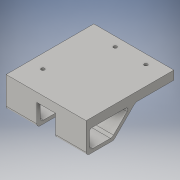
# Autodesk Inventor part: Base
Saved by Autodesk Inventor 2016 (Build 200138000, 138)
## iProperties
Created: 2018-09-18
Part Number: Base
Material: Generic
Document SubType Name: Modeling
Designer: Kyle
Density: 1 g/cm^3
Appearance: Default
Author: Kyle
Autodesk Inventor part; units mm, degrees
ref_plane "YZ Plane" through (0, 0, 0) normal (1, 0, 0) x (0, 1, 0)
ref_plane "XZ Plane" through (0, 0, 0) normal (0, 1, 0) x (-1, 0, 0)
ref_plane "XY Plane" through (0, 0, 0) normal (0, 0, 1) x (1, 0, 0)
sketch "Sketch1" plane through (0, 0, 0) normal (0, 1, 0) x (-1, 0, 0)
  line L0 (-36.5, 40) -> (36.5, 40)
  line L1 (36.5, 40) -> (36.5, -40)
  line L2 (36.5, -40) -> (-36.5, -40)
  line L3 (-36.5, -40) -> (-36.5, 40)
  line L4 (-36.5, 40) -> (36.5, -40) construction
  line L5 (36.5, 40) -> (-36.5, -40) construction
  line L6 (36.5, 40) -> (36.5, 13)
  line L7 (-36.5, -40) -> (-9.5, -40)
  line L8 (-36.5, -40) -> (18.5, -40)
  circle A0 centre (8.5, -31.5) radius 1.5
  circle A1 centre (-19.5, -31.5) radius 1.5
  circle A2 centre (-19.5, -31.5) radius 1.5
  circle A3 centre (24, 19) radius 1.5
  line L9 (0, 0) -> (0, 17.5)
  line L10 (0, 17.5) -> (0, 19)
  line L11 (0, 19) -> (24, 19)
  line L12 (0, 0) -> (0, -31.5)
  line L13 (0, -31.5) -> (8.5, -31.5)
  line L14 (0, -31.5) -> (-19.5, -31.5)
  dimension "d0" = 73
  dimension "d1" = 80
  dimension "d5" = 3
  dimension "d6" = 3
  dimension "d7" = 3
  dimension "d10" = 17.5
  dimension "d11" = 8.5
  dimension "d12" = 19.5
  dimension "d13" = 31.5
  dimension "d14" = 24
  constraints: 30 end point, 5 point on line, 4 centre point, 4 perpendicular, 3 horizontal, 2 midpoint, 2 parallel, 2 vertical, 1 coincident, 1 concentric
  measures "d0" distance of L1.end L3.start
  measures "d1" distance of L1.start L1.end
  measures "d5" diameter of A0
  measures "d6" diameter of A1
  measures "d7" diameter of A3
  measures "d10" distance of L9.start L9.end
  measures "d11" distance of L12.end L13.end
  measures "d12" distance of L12.end L14.end
  measures "d13" distance of L9.start L12.end
  measures "d14" distance of L10.end L11.end
extrude "Extrusion1" add sketch "Sketch1" along normal blind 8
sketch "Sketch2" plane through (36.5, 0, 40) normal (1, 0, 0) x (0, 0, -1)
  line L0 (75, 0) -> (55, 0)
  line L1 (80, 0) -> (0, 0) projected
  line L2 (55, 0) -> (35, 0)
  line L3 (0, 0) -> (32.9289, 0)
  line L4 (44.0711, 0) -> (32.9289, 0)
  line L5 (75, 0) -> (80, 0)
  line L6 (5, 0) -> (25, 0)
  line L7 (23.7574, -20) -> (3, -20)
  line L8 (0, -17) -> (0, 0)
  line L9 (0, 0) -> (80, 0)
  line L10 (22.1005, -17) -> (6, -17)
  line L11 (3, -14) -> (3, -2)
  line L12 (3, -2.5) -> (3, -2)
  line L13 (25, 0) -> (45, 0)
  line L14 (25.8787, -19.1213) -> (43.5355, -1.4645)
  line L15 (24.9289, -15.8284) -> (37.3431, -3.4142)
  arc A0 (22.1005, -17) -> (24.9289, -15.8284) centre (22.1005, -13) ccw
  arc A1 (3, -14) -> (6, -17) centre (6, -14) ccw
  arc A2 (0, -17) -> (3, -20) centre (3, -17) ccw
  arc A3 (23.7574, -20) -> (25.8787, -19.1213) centre (23.7574, -17) ccw
  arc A4 (37.3431, -3.4142) -> (35.9289, 0) centre (35.9289, -2) ccw
  arc A5 (5, 0) -> (3, -2) centre (5, -2) ccw
  line L16 (80, 0) -> (47.0711, 0)
  arc A6 (47.0711, 0) -> (43.5355, -1.4645) centre (47.0711, -5) ccw
  line L17 (35.9289, 0) -> (47.0711, 0)
  line L18 (5, 0) -> (0, 0)
  point P0 (40, 0)
  point P1 (39.2426, 0)
  point P2 (25, -20)
  point P3 (0, -20)
  point P4 (40.7574, 0)
  constraints: 36 end point, 17 point on line, 15 point on circle, 7 centre point, 1 collinear, 1 horizontal, 1 other
extrude "Extrusion3" add sketch "Sketch2" against normal up to surface (73 mm away) contours A6 L14 A3 L7 A2 L8 L1 A5 L11 A1 L10 A0 L15 A4
sketch "Sketch3" plane through (-36.5, 8, 40) normal (0, 0, 1) x (1, 0, 0)
  line L0 (0, 0) -> (28, 0)
  line L1 (0, 0) -> (73, 0) projected
  line L2 (73, 0) -> (45, 0)
  line L3 (73, -28) -> (0, -28) projected
  line L4 (28, 0) -> (45, 0)
  line L5 (45, 0) -> (45, -28)
  line L6 (45, -28) -> (28, -28)
  line L7 (28, -28) -> (28, 0)
  line L8 (73, -8) -> (0, -8) projected
  line L9 (28, 0) -> (45, 0)
  line L10 (45, 0) -> (45, -8)
  line L11 (45, -8) -> (28, -8)
  line L12 (28, -8) -> (28, 0)
  point P0 (36.5, -8)
  dimension "d32" = 28
  dimension "d33" = 28
  constraints: 20 end point, 5 point on line, 4 parallel, 2 horizontal, 2 perpendicular
  measures "d32" distance of L0.start L0.end
  measures "d33" distance of L1.end L2.end
extrude "Extrusion4" cut sketch "Sketch3" against normal up to surface (80 mm away) contours L8 L5 L3 L7
body "Solid1"
